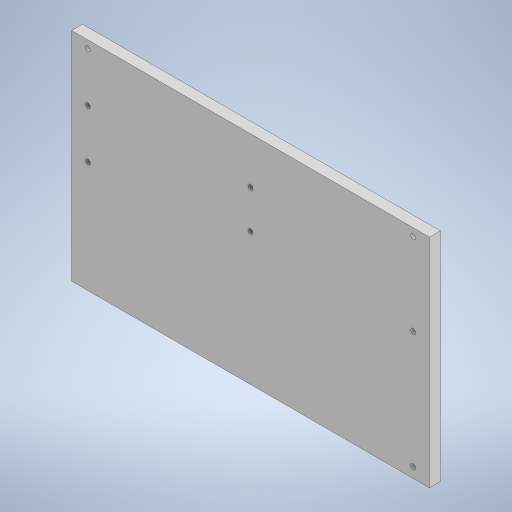
# Autodesk Inventor part: Validation_jig_top
Saved by Autodesk Inventor 2023 (Build 270158000, 158)
## iProperties
Created: 2023-02-22
Part Number: Validation_jig_top
Material: Générique
Document SubType Name: Modeling
Designer: jfcoe
Density: 1 g/cm^3
Appearance: Par défaut
Author: jfcoe
Autodesk Inventor part; units mm, degrees
ref_plane "YZ Plane" through (0, 0, 0) normal (1, 0, 0) x (0, 1, 0)
ref_plane "XZ Plane" through (0, 0, 0) normal (0, 1, 0) x (-1, 0, 0)
ref_plane "XY Plane" through (0, 0, 0) normal (0, 0, 1) x (1, 0, 0)
sketch "Esquisse1" plane through (0, 0, 0) normal (0, 0, 1) x (1, 0, 0)
  line L0 (0, 0) -> (220, 0)
  line L1 (220, 0) -> (220, -133.5)
  line L2 (220, -133.5) -> (0, -133.5)
  line L3 (0, -133.5) -> (0, 0)
  dimension "d0" = 220
  dimension "d1" = 133.5
  constraints: 8 end point, 2 parallel, 1 horizontal, 1 perpendicular
  measures "d0" distance of L1.end L2.end
  measures "d1" distance of L0.end L1.end
extrude "Extrusion1" add sketch "Esquisse1" against normal blind 6.7
sketch "Esquisse2" plane through (0, 0, 0) normal (0, 0, 1) x (1, 0, 0)
  circle A0 centre (10, -4.675) radius 1.524
  circle A1 centre (10, -35) radius 1.524
  circle A2 centre (10, -65) radius 1.524
  circle A3 centre (110, -28.5) radius 1.524
  circle A4 centre (110, -52) radius 1.524
  circle A5 centre (210, -4.675) radius 1.524
  circle A6 centre (210, -55.175) radius 1.524
  circle A7 centre (210, -127.175) radius 1.524
  line L0 (0, 0) -> (0, -133.5) projected
  line L1 (220, 0) -> (0, 0) projected
  line L2 (220, -133.5) -> (220, 0) projected
  dimension "d4" = 3.048
  dimension "d5" = 10
  dimension "d6" = 4.675
  dimension "d7" = 4.675
  dimension "d8" = 10
  dimension "d9" = 10
  dimension "d10" = 10
  dimension "d13" = 10
  dimension "d14" = 10
  dimension "d15" = 30
  dimension "d16" = 30.325
  dimension "d17" = 50.5
  dimension "d18" = 72
  dimension "d19" = 28.5
  dimension "d20" = 23.5
  dimension "d23" = 110
  dimension "d24" = 110
  constraints: 8 centre point, 7 equal radius
  measures "d4" diameter of A0
  measures "d5" distance from line of L0 A0.centre
  measures "d6" distance from line of L1 A0.centre
  measures "d7" distance from line of L1 A5.centre
  measures "d8" distance from line of L2 A5.centre
  measures "d9" distance from line of L2 A6.centre
  measures "d10" distance from line of L2 A7.centre
  measures "d13" distance from line of L0 A1.centre
  measures "d14" distance from line of L0 A2.centre
  measures "d15" distance of A2.centre A1.centre
  measures "d16" distance of A1.centre A0.centre
  measures "d17" distance of A6.centre A5.centre
  measures "d18" distance of A7.centre A6.centre
  measures "d19" distance from line of L1 A3.centre
  measures "d20" distance of A4.centre A3.centre
  measures "d23" distance from line of L0 A3.centre
  measures "d24" distance from line of L0 A4.centre
extrude "Extrusion2" cut sketch "Esquisse2" against normal through all
